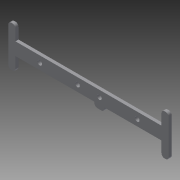
# Autodesk Inventor part: OuterBar
Saved by Autodesk Inventor 2014 SP1 (Build 180222100, 222)
## iProperties
Created: 2014-06-07
Part Number: OuterBar
Material: Generic
Document SubType Name: Modeling
Designer: Erin
Density: 1 g/cm^3
Appearance: Default
Author: Erin
Autodesk Inventor part; units mm, degrees
ref_plane "YZ Plane" through (0, 0, 0) normal (1, 0, 0) x (0, 1, 0)
ref_plane "XZ Plane" through (0, 0, 0) normal (0, 1, 0) x (-1, 0, 0)
ref_plane "XY Plane" through (0, 0, 0) normal (0, 0, 1) x (1, 0, 0)
sketch "Sketch1" plane through (0, 0, 0) normal (0, 1, 0) x (-1, 0, 0)
  line L0 (-75.4, 6.25) -> (75.4, 6.25)
  line L1 (78.4, 3.25) -> (78.4, -3.25)
  line L2 (75.4, -6.25) -> (-75.4, -6.25)
  line L3 (-78.4, -3.25) -> (-78.4, 3.25)
  circle A0 centre (-47.65, 0) radius 2.25
  circle A1 centre (47.65, 0) radius 2.25
  circle A2 centre (-47.65, 0) radius 26.75 construction
  circle A3 centre (-10.7, 0) radius 2.25
  circle A4 centre (-10.7, 0) radius 11.2 construction
  line L4 (-21.9, 0) -> (-21.9, 5.3604)
  line L5 (-20.9, 0) -> (-20.9, 5.3604)
  circle A5 centre (10.7, 0) radius 2.25
  circle A6 centre (10.7, 0) radius 11.2 construction
  line L6 (-0.5, 0) -> (-0.5, 4.194)
  line L7 (0.5, 0) -> (0.5, 4.194)
  circle A7 centre (47.65, 0) radius 26.75 construction
  line L8 (20.9, 0) -> (20.9, 4.3426)
  line L9 (21.9, 0) -> (21.9, 4.3426)
  arc A8 (-75.4, 6.25) -> (-78.4, 3.25) centre (-75.4, 3.25) ccw
  arc A9 (-78.4, -3.25) -> (-75.4, -6.25) centre (-75.4, -3.25) ccw
  arc A10 (78.4, 3.25) -> (75.4, 6.25) centre (75.4, 3.25) ccw
  arc A11 (75.4, -6.25) -> (78.4, -3.25) centre (75.4, -3.25) ccw
  line L10 (-81.9483, 0) -> (80.5332, 0) construction
  line L11 (-15.7, 6.25) -> (-5.7, 6.25)
  line L12 (-15.7, -6.25) -> (-5.7, -6.25)
  line L13 (-5.7, -6.25) -> (-5.7, -7.25)
  line L14 (-8.7, -10.25) -> (-12.7, -10.25)
  line L15 (-15.7, -7.25) -> (-15.7, -6.25)
  arc A12 (-15.7, -7.25) -> (-12.7, -10.25) centre (-12.7, -7.25) ccw
  arc A13 (-8.7, -10.25) -> (-5.7, -7.25) centre (-8.7, -7.25) ccw
  line L16 (74.4, 0) -> (74.4, 9.25)
  line L17 (-74.4, 0) -> (-74.4, 10.75)
  line L18 (-75.4, 20) -> (-74.4, 20)
  line L19 (-71.4, 17) -> (-71.4, -17)
  line L20 (-74.4, -20) -> (-75.4, -20)
  line L21 (-78.4, -17) -> (-78.4, 17)
  line L22 (75.4, 20) -> (74.4, 20)
  line L23 (71.4, 17) -> (71.4, -17)
  line L24 (74.4, -20) -> (75.4, -20)
  line L25 (78.4, -17) -> (78.4, 17)
  arc A14 (-75.4, 20) -> (-78.4, 17) centre (-75.4, 17) ccw
  arc A15 (-71.4, 17) -> (-74.4, 20) centre (-74.4, 17) ccw
  arc A16 (-78.4, -17) -> (-75.4, -20) centre (-75.4, -17) ccw
  arc A17 (-74.4, -20) -> (-71.4, -17) centre (-74.4, -17) ccw
  arc A18 (74.4, 20) -> (71.4, 17) centre (74.4, 17) ccw
  arc A19 (78.4, 17) -> (75.4, 20) centre (75.4, 17) ccw
  arc A20 (75.4, -20) -> (78.4, -17) centre (75.4, -17) ccw
  arc A21 (71.4, -17) -> (74.4, -20) centre (74.4, -17) ccw
  line L26 (-18.7, 7.9059) -> (-18.7, -10.25)
  line L27 (-2.7, 9.25) -> (-2.7, -10.25)
  point P0 (0, 0)
  point P1 (-78.4, 6.25)
  point P2 (-78.4, -6.25)
  point P3 (0, 6.25)
  point P4 (78.4, 0)
  point P5 (-78.4, 20)
  point P6 (-71.4, 20)
  point P7 (-78.4, -20)
  point P8 (-71.4, 0)
  point P9 (-78.4, 0)
  point P10 (78.4, 20)
  point P11 (71.4, 20)
  point P12 (78.4, -20)
  point P13 (78.4, 0)
  dimension "d0" = 12.5
  dimension "d1" = 4.5
  dimension "d3" = 4.5
  dimension "d5" = 53.5
  dimension "d6" = 4.5
  dimension "d7" = 22.4
  dimension "d8" = 1
  dimension "d9" = 4.5
  dimension "d10" = 22.4
  dimension "d11" = 1
  dimension "d12" = 53.5
  dimension "d13" = 1
  dimension "d14" = 3
  dimension "d29" = 4
  dimension "d30" = 148.8
  dimension "d31" = 4
  dimension "d32" = 7
  dimension "d33" = 40
  dimension "d34" = 7
  dimension "d35" = 40
  dimension "d36" = 3
  dimension "d37" = 3
  dimension "d39" = 3
  dimension "d40" = 3
  dimension "d42" = 1
  dimension "d43" = 8
  dimension "d44" = 8
  dimension "d45" = 16
  constraints: 56 end point, 36 point on circle, 32 tangent, 22 centre point, 20 point on line, 16 parallel, 9 equal radius, 5 coincident, 5 horizontal, 5 midpoint, 4 perpendicular, 2 collinear, 2 horizontal alignment, 2 symmetric about line, 1 vertical alignment
  measures "d0" distance of point (-78.4, -6.25) point (-78.4, 6.25)
  measures "d1" diameter of A0
  measures "d3" diameter of A1
  measures "d5" diameter of A2
  measures "d6" diameter of A3
  measures "d7" diameter of A4
  measures "d8" distance between parallel lines of L5 L4
  measures "d9" diameter of A5
  measures "d10" diameter of A6
  measures "d11" distance between parallel lines of L7 L6
  measures "d12" diameter of A7
  measures "d13" distance between parallel lines of L9 L8
  measures "d14" radius of A8
  measures "d29" distance between parallel lines of L16 L1
  measures "d30" distance between parallel lines of L16 L17
  measures "d31" distance between parallel lines of L3 L17
  measures "d32" distance of point (-78.4, 20) point (-71.4, 20)
  measures "d33" distance of point (-78.4, -20) point (-78.4, 20)
  measures "d34" distance of point (78.4, 20) point (71.4, 20)
  measures "d35" distance of point (78.4, -20) point (78.4, 20)
  measures "d36" radius of A14
  measures "d37" radius of A18
  measures "d39" radius of A13
  measures "d40" radius of A12
  measures "d42" distance of L15.start L12.start
  measures "d43" distance from line of A3.centre L27
  measures "d44" distance from line of A3.centre L26
  measures "d45" distance between parallel lines of L27 L26
extrude "Extrusion1" add sketch "Sketch1" along normal blind 3
chamfer "Chamfer2" [suppressed]
body "Solid1"
